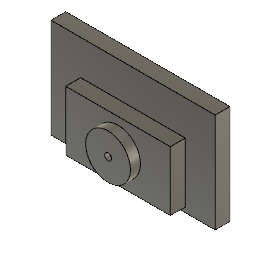
Kamera v2 (Autodesk Fusion 360 design; units mm, degrees)
Autodesk Fusion 360 part; units mm, degrees
box "BoxPrimitive1" add length 20 width 33 height 3 placed x (0, 0, 1) y (1, 0, 0) z (0, 1, 0) at (0, 0, 0)
sketch "Sketch2" plane through (0, 0, 0) normal (0, -1, 0) x (1, 0, 0)
  line L0 (33, 20) -> (0, 20)
  line L1 (0, 20) -> (0, 0)
  line L2 (0, 0) -> (33, 0)
  line L3 (33, 0) -> (33, 20)
  line L4 (16.5, 20) -> (16.5, 0)
  line L5 (16.5, 0) -> (16.5, 1)
  line L6 (16.5, 1) -> (27, 1)
  line L7 (27, 1) -> (6, 1)
  line L8 (6, 1) -> (6, 13)
  line L9 (6, 13) -> (27, 13)
  line L10 (27, 13) -> (27, 1)
  dimension "d6" = 1
  dimension "d7" = 10.5
  dimension "d8" = 21
  dimension "d9" = 12
  constraint midpoint L0 L4.start
  constraint midpoint L2 L4.end
  constraint vertical L5
  constraint perpendicular L5 L6
  constraint horizontal L7
  constraint vertical L8
  constraint horizontal L9
  constraint vertical L10
  measures "d6" distance of L4.end L5.end
  measures "d7" distance of L5.end L6.end
  measures "d8" distance of L6.end L7.end
  measures "d9" distance of L6.end L9.end
extrude "Extrude1" add sketch "Sketch2" along normal blind 3 contours L4 L6 L7 L9 L10 | L4 L7 L8 L9
sketch "Sketch3" plane through (0, -3, 0) normal (0, -1, 0) x (1, 0, 0)
  line L0 (27, 13) -> (6, 13)
  line L1 (6, 13) -> (6, 1)
  line L2 (6, 1) -> (27, 1)
  line L3 (27, 1) -> (27, 13)
  line L4 (16.5, 13) -> (16.5, 1)
  line L5 (6, 7) -> (27, 7)
  constraint midpoint L0 L4.start
  constraint midpoint L2 L4.end
  constraint midpoint L1 L5.start
  constraint midpoint L3 L5.end
cylinder "CylinderPrimitive1" add diameter 9 height 2 placed x (1, 0, 0) y (0, 0, 1) z (0, -1, 0) at (16.5, -3, 7)
cylinder "CylinderPrimitive2" cut diameter 1.37 height -2 placed x (1, 0, 0) y (0, 0, 1) z (0, -1, 0) at (16.5, -5, 7)
